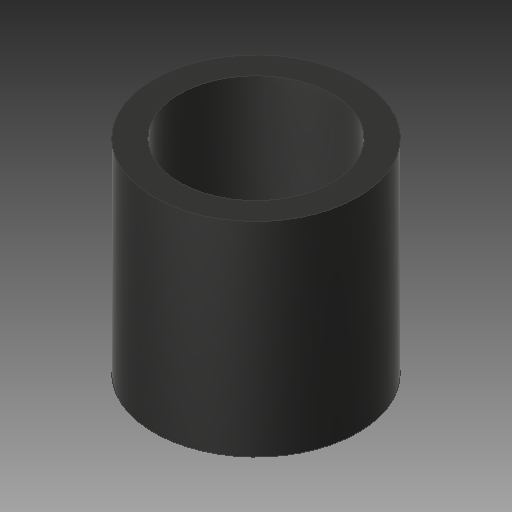
# Autodesk Inventor part: オイレス060808
Saved by Autodesk Inventor 2019 (Build 230136000, 136)
## iProperties
Part Number: オイレス060808
Material: 一般
Document SubType Name: Modeling
Designer: 雪村
Density: 1 g/cm^3
Appearance: 滑らか - 黒
Mass: 0.175929 g
Surface Area: 3.95841 cm^2
Volume: 0.175929 cm^3
Author: 雪村
Autodesk Inventor part; units mm, degrees
ref_plane "YZ Plane" through (0, 0, 0) normal (1, 0, 0) x (0, 1, 0)
ref_plane "XZ Plane" through (0, 0, 0) normal (0, 1, 0) x (-1, 0, 0)
ref_plane "XY Plane" through (0, 0, 0) normal (0, 0, 1) x (1, 0, 0)
sketch "スケッチ1" plane through (0, 0, 0) normal (0, 1, 0) x (-1, 0, 0)
  circle A0 centre (0, 0) radius 3
  circle A1 centre (0, 0) radius 4
  dimension "d0" = 6
  dimension "d1" = 8
  constraints: 2 centre point, 2 coincident
  measures "d0" diameter of A0
  measures "d1" diameter of A1
extrude "押し出し1" add sketch "スケッチ1" along normal blind 8
